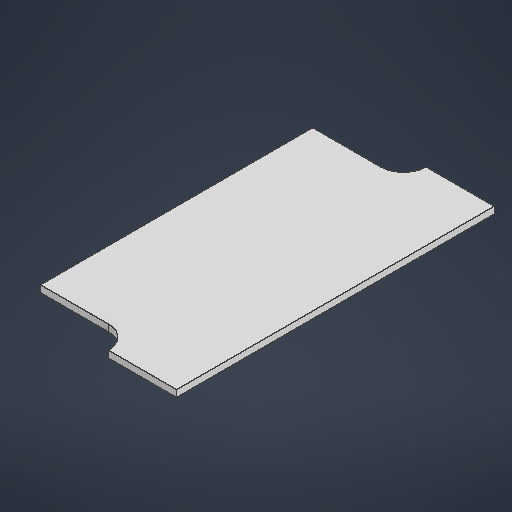
# Autodesk Inventor part: lateral_base
Saved by Autodesk Inventor 2026.1 (Build 301233000, 233)
## iProperties
Created: 2025-10-15
Part Number: lateral_base
Material: Generic
Document SubType Name: Modeling
Designer: emanuel
Density: 1 g/cm^3
Appearance: Default
Author: emanuel
Autodesk Inventor part; units mm, degrees
ref_plane "YZ Plane" through (0, 0, 0) normal (1, 0, 0) x (0, 1, 0)
ref_plane "XZ Plane" through (0, 0, 0) normal (0, 1, 0) x (-1, 0, 0)
ref_plane "XY Plane" through (0, 0, 0) normal (0, 0, 1) x (1, 0, 0)
sketch "Sketch1" plane through (0, 0, 0) normal (0, 1, 0) x (-1, 0, 0)
  line L0 (0, 0) -> (-30, 0)
  line L1 (-30, 0) -> (-30, -140)
  line L2 (-30, -140) -> (0, -140)
  line L3 (0, -140) -> (0, 0)
  line L4 (0, 0) -> (0, -10)
  line L5 (0, -10) -> (40, -10)
  line L6 (40, -10) -> (40, -130)
  line L7 (40, -130) -> (0, -130)
  line L8 (0, -130) -> (0, -10)
  point P0 (0, -130)
  dimension "d0" = 30
  dimension "d1" = 140
  dimension "d2" = 10
  dimension "d3" = 40
  dimension "d4" = 120
  constraints: 18 end point, 4 parallel, 2 horizontal, 2 perpendicular, 1 point on line
  measures "d0" distance of L2.end L1.end
  measures "d1" distance of L1.end L0.end
  measures "d2" distance of L0.start L4.end
  measures "d3" distance of L6.end L7.end
  measures "d4" distance of L5.end L6.end
extrude "Extrusion1" add sketch "Sketch1" along normal blind 3
fillet "Fillet1" radius 10 2 edges at (0, 1.5, -10) (0, 1.5, -130)
body "Solid1"
